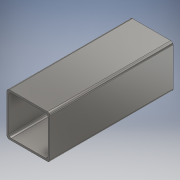
# Autodesk Inventor part: AlignmentTube
Saved by Autodesk Inventor 2018 (Build 220112000, 112)
## iProperties
Created: 2017-10-24
Part Number: AlignmentTube
Material: Steel, Mild
Document SubType Name: Modeling
Designer: P136265
Density: 7.85 g/cm^3
Appearance: Semi-Polished
Mass: 167.802 g
Surface Area: 264.608 cm^2
Volume: 21.376 cm^3
Author: P136265
Autodesk Inventor part; units mm, degrees
ref_plane "YZ Plane" through (0, 0, 0) normal (1, 0, 0) x (0, 1, 0)
ref_plane "XZ Plane" through (0, 0, 0) normal (0, 1, 0) x (-1, 0, 0)
ref_plane "XY Plane" through (0, 0, 0) normal (0, 0, 1) x (1, 0, 0)
sketch "Sketch1" plane through (0, 0, 0) normal (0, 1, 0) x (-1, 0, 0)
  line L0 (-15.5, 17.5) -> (15.5, 17.5)
  line L1 (17.5, 15.5) -> (17.5, -15.5)
  line L2 (15.5, -17.5) -> (-15.5, -17.5)
  line L3 (-17.5, -15.5) -> (-17.5, 15.5)
  line L4 (-17.5, 17.5) -> (17.5, -17.5) construction
  line L5 (17.5, 17.5) -> (-17.5, -17.5) construction
  line L6 (-13.9, -15.9) -> (13.9, -15.9)
  line L7 (15.9, -13.9) -> (15.9, 13.9)
  line L8 (13.9, 15.9) -> (-13.9, 15.9)
  line L9 (-15.9, 13.9) -> (-15.9, -13.9)
  arc A0 (17.5, 15.5) -> (15.5, 17.5) centre (15.5, 15.5) ccw
  arc A1 (15.5, -17.5) -> (17.5, -15.5) centre (15.5, -15.5) ccw
  arc A2 (-17.5, -15.5) -> (-15.5, -17.5) centre (-15.5, -15.5) ccw
  arc A3 (-15.5, 17.5) -> (-17.5, 15.5) centre (-15.5, 15.5) ccw
  arc A4 (15.9, 13.9) -> (13.9, 15.9) centre (13.9, 13.9) ccw
  arc A5 (13.9, -15.9) -> (15.9, -13.9) centre (13.9, -13.9) ccw
  arc A6 (-15.9, -13.9) -> (-13.9, -15.9) centre (-13.9, -13.9) ccw
  arc A7 (-13.9, 15.9) -> (-15.9, 13.9) centre (-13.9, 13.9) ccw
  point P0 (0, 0)
  dimension "d0" = 35
  dimension "d1" = 35
  dimension "d2" = 1.6
  dimension "d3" = 2
  constraints: 20 end point, 16 point on circle, 16 tangent, 8 centre point, 8 point on line, 7 equal radius, 4 parallel, 2 midpoint, 2 perpendicular, 1 horizontal, 3 other
  measures "d0" distance of L4.end L5.end
  measures "d1" distance of L5.start L4.end
  measures "d2" distance between parallel lines of L2 L6
  measures "d3" radius of A0
extrude "Extrusion1" add sketch "Sketch1" along normal blind 100
body "Solid1"
